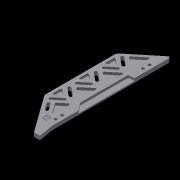
# Autodesk Inventor part: HipShockPlateRight
Saved by Autodesk Inventor 2015 (Build 190159000, 159)
## iProperties
RuleStatus: InUse
Created: 2014-08-28
Part Number: HipShockPlateRight
Material: Generic
Document SubType Name: Modeling
Designer: Inventor
Density: 1 g/cm^3
Appearance: Default
Mass: 78.3969 g
Surface Area: 353.49 cm^2
Volume: 78.3969 cm^3
BeforeDocSave0: UpdateBoundingBox
CX: 66.60 mm
CY: 268.39 mm
CZ: 8.00 mm
Author: Inventor
Autodesk Inventor part; units mm, degrees
ref_plane "YZ Plane" through (0, 0, 0) normal (1, 0, 0) x (0, 1, 0)
ref_plane "XZ Plane" through (0, 0, 0) normal (0, 1, 0) x (-1, 0, 0)
sketch "Base" plane through (0, 0, 0) normal (0, 0, 1) x (1, 0, 0)
  line L0 (6.9563, 266) -> (3.8969, 268.7067)
  line L1 (-54.5437, 220.9056) -> (3.8969, 268.7067)
  line L2 (-54.5437, 220.9056) -> (-54.5437, 75.9056)
  line L3 (0, 0) -> (12.2461, 0)
  line L4 (0, 0) -> (-54.5437, 75.9056)
  line L5 (6.9563, 30) -> (12.2461, 0)
  line L6 (6.9563, 266) -> (6.9563, 30)
  dimension "d1" = 170
  dimension "d3" = 131.5
  dimension "d4" = 99.219
  dimension "d5" = 75.5
  dimension "d6" = 145
  dimension "d7" = 129.281
  dimension "d8" = 144.3
  dimension "d9" = 125.7
  dimension "d10" = 236
  dimension "d11" = 30
  dimension "d15" = 61.5
  constraints: 14 end point, 1 coincident, 1 horizontal, 1 parallel, 1 vertical
  measures "d1" angle of L6 L5
  measures "d3" angle of L0 L6
  measures "d4" angle of L1 L0
  measures "d5" distance of L1.start L0.end
  measures "d6" distance of L1.start L2.end
  measures "d7" angle of L2 L1
  measures "d8" angle of L2 L4
  measures "d9" angle of L4 L3
  measures "d10" distance of L0.start L5.start
  measures "d11" vertical distance of L5.start L3.end
  measures "d15" distance between parallel lines of L6 L2
extrude "BaseFeature" add sketch "Base" along normal blind 8
fillet "BaseFillet1Feature" radius 9 1 edges at (-54.5437, 220.9056, 4)
fillet "BaseFillet2Feature" radius 6 1 edges at (-54.5437, 75.9056, 4)
ref_plane "BaseTopPlane" through (0, 0, 8) normal (0, 0, 1) x (1, 0, 0)
sketch "InsetDetail" plane through (0, 0, 8) normal (0, 0, 1) x (1, 0, 0)
  line L0 (-12.0437, 248.5627) -> (-12.0437, 208.0737)
  line L1 (-12.0437, 208.0737) -> (-36.7942, 228.3182)
  line L2 (-36.7942, 228.3182) -> (-12.0437, 248.5627)
  line L3 (-34.9841, 201.5737) -> (-49.0437, 190.0737)
  line L4 (-49.0437, 213.0737) -> (-34.9841, 201.5737)
  line L5 (-49.0437, 190.0737) -> (-49.0437, 213.0737)
  line L6 (-36.5437, 175.0341) -> (-12.0437, 195.0737)
  line L7 (-12.0437, 195.0737) -> (-12.0437, 154.5847)
  line L8 (-12.0437, 154.5847) -> (-36.5437, 175.0341)
  line L9 (-35.2658, 148.0847) -> (-49.0437, 136.5847)
  line L10 (-49.0437, 159.5847) -> (-35.2658, 148.0847)
  line L11 (-49.0437, 136.5847) -> (-49.0437, 159.5847)
  line L12 (-36.2982, 121.3402) -> (-12.0437, 141.5847)
  line L13 (-12.0437, 141.5847) -> (-12.0437, 101.0957)
  line L14 (-12.0437, 101.0957) -> (-36.2982, 121.3402)
  line L15 (-35.2658, 94.5957) -> (-49.0437, 83.0957)
  line L16 (-49.0437, 106.0957) -> (-35.2658, 94.5957)
  line L17 (-49.0437, 83.0957) -> (-49.0437, 106.0957)
  line L18 (-30.2303, 72.916) -> (-12.0437, 47.6068)
  line L19 (-12.0437, 88.0957) -> (-12.0437, 47.6068)
  line L20 (-30.2303, 72.916) -> (-12.0437, 88.0957)
  line L21 (-5.0437, 98.1402) -> (-5.0437, 194.9501)
  line L22 (6.9563, 196) -> (-5.0437, 194.9501)
  line L23 (6.9563, 83) -> (-5.0437, 98.1402)
  line L24 (6.9563, 30) -> (6.9563, 266) construction
  line L25 (6.9563, 196) -> (6.9563, 83)
  line L26 (-54.5437, 216.6399) -> (-54.5437, 77.8378) construction
  line L27 (3.8969, 268.7067) -> (-51.2419, 223.6064) construction
  line L28 (-53.4162, 74.3365) -> (0, 0) construction
  line L29 (-49.0437, 201.5737) -> (6.9563, 201.5737) construction
  line L30 (-49.0437, 148.0847) -> (6.9563, 148.0847) construction
  line L31 (-49.0437, 94.5957) -> (6.9563, 94.5957) construction
  line L32 (-36.7942, 228.3182) -> (-12.0437, 228.3182) construction
  line L33 (-36.5437, 175.0341) -> (-12.0437, 175.0341) construction
  line L34 (-36.2982, 121.3402) -> (-12.0437, 121.3402) construction
  line L35 (-30.2303, 72.916) -> (-12.0437, 72.916) construction
  dimension "d21" = 95
  dimension "d22" = 141.6
  dimension "d23" = 12
  dimension "d24" = 113
  dimension "d25" = 70
  dimension "d27" = 5.5
  dimension "d29" = 5.5
  dimension "d30" = 5.5
  dimension "d66" = 13
  dimension "d67" = 13
  dimension "d90" = 18
  dimension "d91" = 6.5
  dimension "d93" = 6.5
  dimension "d94" = 6.5
  dimension "d95" = 13
  dimension "d97" = 19
  dimension "d98" = 19
  dimension "d99" = 19
  dimension "d100" = 19
  dimension "d102" = 5.5
  dimension "d105" = 23
  dimension "d106" = 18
  constraints: 64 end point, 16 parallel, 10 point on line, 6 perpendicular, 5 collinear, 5 midpoint, 1 horizontal, 1 vertical
  measures "d21" angle of L22 L21
  measures "d22" angle of L21 L23
  measures "d23" distance between parallel lines of L21 L24
  measures "d24" distance of L23.start L22.start
  measures "d25" distance of L22.start L24.end
  measures "d27" distance between parallel lines of L27 L2
  measures "d29" distance between parallel lines of L26 L11
  measures "d30" distance between parallel lines of L26 L17
  measures "d66" distance of L6.end L0.end
  measures "d67" distance of L12.end L7.end
  measures "d90" distance between parallel lines of L28 L18
  measures "d91" distance from line of L29 L0.end
  measures "d93" distance from line of L30 L7.end
  measures "d94" distance from line of L31 L13.end
  measures "d95" distance of L19.start L13.end
  measures "d97" distance between parallel lines of L24 L0
  measures "d98" distance between parallel lines of L24 L7
  measures "d99" distance between parallel lines of L24 L13
  measures "d100" distance between parallel lines of L24 L19
  measures "d102" distance between parallel lines of L26 L5
  measures "d105" distance of L9.end L10.start
  measures "d106" distance from line of L26 L6.start
extrude "InsetsFeature" cut sketch "InsetDetail" against normal blind 5
fillet "InsetFillet1Feature" radius 3 1 edges at (-5.0437, 194.9501, 5.5)
fillet "InsetFillet2Feature" radius 4 1 edges at (-5.0437, 98.1402, 5.5)
fillet "TriangleInsetFilletsFeature" radius 2 21 edges at (-12.0437, 248.5627, 5.5) (-36.7942, 228.3182, 5.5) (-12.0437, 208.0737, 5.5) (-12.0437, 154.5847, 5.5) (-36.5437, 175.0341, 5.5) (-12.0437, 195.0737, 5.5) (-49.0437, 213.0737, 5.5) (-49.0437, 190.0737, 5.5) (-34.9841, 201.5737, 5.5) (-49.0437, 136.5847, 5.5) (-49.0437, 159.5847, 5.5) (-35.2658, 148.0847, 5.5) (-12.0437, 141.5847, 5.5) (-36.2982, 121.3402, 5.5) (-12.0437, 101.0957, 5.5) (-49.0437, 106.0957, 5.5) (-49.0437, 83.0957, 5.5) (-35.2658, 94.5957, 5.5) (-30.2303, 72.916, 5.5) (-12.0437, 88.0957, 5.5) (-12.0437, 47.6068, 5.5)
sketch "VariableHoles" plane through (0, 0, 8) normal (0, 0, 1) x (1, 0, 0)
  line L0 (-45.7775, 210.4021) -> (-36.8767, 203.1218) construction
  line L1 (-15.31, 210.7453) -> (-34.9015, 226.7701) construction
  line L2 (-36.8767, 200.0256) -> (-45.7775, 192.7453) construction
  line L3 (-34.4587, 122.8757) -> (-15.3253, 138.8457) construction
  line L4 (-45.7621, 103.3567) -> (-37.1054, 96.1312) construction
  line L5 (-15.3253, 103.8348) -> (-34.4587, 119.8048) construction
  line L6 (-37.1054, 93.0603) -> (-45.7621, 85.8348) construction
  line L7 (-28.8022, 74.108) -> (-15.3253, 85.3567) construction
  line L8 (-15.6679, 52.6503) -> (-29.1448, 71.4054) construction
  line L9 (-53.4162, 74.3365) -> (0, 0) construction
  line L10 (-42.1468, 220.0644) -> (-26.6658, 207.4018) construction
  line L11 (6.9563, 30) -> (6.9563, 266) construction
  arc A0 (-28.5652, 205.0797) -> (-24.7665, 209.724) centre (-26.6658, 207.4018) ccw
  arc A1 (-40.2474, 222.3865) -> (-44.0462, 217.7422) centre (-42.1468, 220.0644) ccw
  line L12 (-40.2474, 222.3865) -> (-24.7665, 209.724)
  line L13 (-44.0462, 217.7422) -> (-28.5652, 205.0797)
  line L14 (3.8969, 268.7067) -> (-51.2419, 223.6064) construction
  line L15 (-34.9015, 229.8663) -> (-15.31, 245.8911) construction
  line L16 (-49.0437, 194.2934) -> (-49.0437, 208.854) construction
  line L17 (-49.0437, 201.5737) -> (6.9563, 201.5737) construction
  line L18 (-42.1468, 183.0831) -> (-26.6658, 195.7456) construction
  arc A2 (-24.7665, 193.4235) -> (-28.5652, 198.0677) centre (-26.6658, 195.7456) ccw
  arc A3 (-44.0462, 185.4052) -> (-40.2474, 180.7609) centre (-42.1468, 183.0831) ccw
  line L19 (-40.2474, 180.7609) -> (-24.7665, 193.4235)
  line L20 (-44.0462, 185.4052) -> (-28.5652, 198.0677)
  line L21 (-54.5437, 216.6399) -> (-54.5437, 77.8378) construction
  line L22 (6.9563, 196) -> (6.9563, 83) projected
  line L23 (-54.5437, 148.0847) -> (6.9563, 148.0847) construction
  line L24 (-54.5437, 175.0284) -> (6.9563, 175.0284) construction
  arc A4 (-34.6701, 176.5666) -> (-34.6855, 173.4831) centre (-33.4039, 175.0185) ccw construction
  arc A5 (-40.2474, 169.296) -> (-44.0462, 164.6517) centre (-42.1468, 166.9738) ccw
  line L25 (-44.0462, 164.6517) -> (-28.5652, 151.9891)
  line L26 (-40.2474, 169.296) -> (-24.7665, 156.6334)
  arc A6 (-28.5652, 151.9891) -> (-24.7665, 156.6334) centre (-26.6658, 154.3113) ccw
  line L27 (-42.1468, 166.9738) -> (-26.6658, 154.3113) construction
  arc A7 (-37.1054, 146.5493) -> (-37.1054, 149.6202) centre (-38.387, 148.0847) ccw construction
  line L28 (-44.0462, 131.5178) -> (-28.5652, 144.1803)
  arc A8 (-24.7665, 139.536) -> (-28.5652, 144.1803) centre (-26.6658, 141.8582) ccw
  line L29 (-40.2474, 126.8735) -> (-24.7665, 139.536)
  arc A9 (-44.0462, 131.5178) -> (-40.2474, 126.8735) centre (-42.1468, 129.1956) ccw
  line L30 (-42.1468, 129.1956) -> (-26.6658, 141.8582) construction
  line L31 (-54.5437, 121.3402) -> (6.9563, 121.3402) construction
  arc A10 (-34.4587, 122.8757) -> (-34.4587, 119.8048) centre (-33.1771, 121.3402) ccw construction
  line L32 (-44.0462, 111.1627) -> (-28.5652, 98.5002)
  arc A11 (-40.2474, 115.807) -> (-44.0462, 111.1627) centre (-42.1468, 113.4849) ccw
  line L33 (-40.2474, 115.807) -> (-24.7665, 103.1445)
  arc A12 (-28.5652, 98.5002) -> (-24.7665, 103.1445) centre (-26.6658, 100.8223) ccw
  line L34 (-42.1468, 113.4849) -> (-26.6658, 100.8223) construction
  line L35 (-54.5437, 94.5957) -> (6.9563, 94.5957) construction
  line L36 (6.9563, 30) -> (6.9563, 83) construction
  arc A13 (-37.1054, 93.0603) -> (-37.1054, 96.1312) centre (-38.387, 94.5957) ccw construction
  line L37 (-44.0462, 78.0288) -> (-28.5652, 90.6913)
  arc A14 (-44.0462, 78.0288) -> (-40.2474, 73.3845) centre (-42.1468, 75.7066) ccw
  line L38 (-42.1468, 75.7066) -> (-26.6658, 88.3692) construction
  line L39 (-40.2474, 73.3845) -> (-24.7665, 86.047)
  arc A15 (-24.7665, 86.047) -> (-28.5652, 90.6913) centre (-26.6658, 88.3692) ccw
  line L40 (-37.8435, 62.9469) -> (-29.0904, 50.7656)
  arc A16 (-32.971, 66.4481) -> (-37.8435, 62.9469) centre (-35.4073, 64.6975) ccw
  line L41 (-35.4073, 64.6975) -> (-26.6541, 52.5162) construction
  line L42 (-32.971, 66.4481) -> (-24.2179, 54.2669)
  arc A17 (-29.0904, 50.7656) -> (-24.2179, 54.2669) centre (-26.6541, 52.5162) ccw
  line L43 (-28.8022, 74.108) -> (-44.0855, 61.3515) construction
  point P0 (-35.4039, 175.0284)
  point P1 (-36.387, 148.0847)
  point P2 (-35.1771, 121.3402)
  point P3 (-36.387, 94.5957)
  point P4 (-37.1579, 67.1337)
  dimension "d81" = 19.5555
  dimension "d82" = 9.7777
  dimension "d83" = 20
  dimension "d85" = 6
  dimension "d86" = 6
  dimension "d87" = 5.5
  dimension "d88" = 8.5
  dimension "d112" = 18
  dimension "d113" = 9
  dimension "d114" = 3
  dimension "d115" = 20
  dimension "d116" = 15
  constraints: 54 end point, 40 symmetric about line, 33 point on circle, 15 point on line, 14 centre point, 14 coincident, 7 tangent, 4 parallel, 4 perpendicular, 1 collinear, 1 horizontal, 1 midpoint, 10 other
  measures "d81" distance between parallel lines of L1 L0
  measures "d82" distance between parallel lines of L1 L10
  measures "d83" distance of L10.start L10.end
  measures "d85" diameter of A0
  measures "d86" diameter of A1
  measures "d87" distance between parallel lines of L14 L15
  measures "d88" distance from line of L14 A1.centre
  measures "d112" distance between parallel lines of L9 L8
  measures "d113" distance between parallel lines of L41 L8
  measures "d114" radius of A17
  measures "d115" distance of L38.start L38.end
  measures "d116" distance of L41.start L41.end
extrude "VariableHolesFeature" cut sketch "VariableHoles" against normal through all
sketch "ConnectorHoles" plane through (0, 0, 8) normal (0, 0, 1) x (1, 0, 0)
  line L0 (-1.0437, 234) -> (-1.0437, 45) construction
  line L1 (-5.0437, 99.5332) -> (-5.0437, 192.2011) construction
  line L2 (6.9563, 30) -> (6.9563, 266) construction
  line L3 (0, 0) -> (12.2461, 0) construction
  point P0 (-1.0437, 221)
  point P1 (-1.0437, 58)
  dimension "d118" = 8
  dimension "d119" = 13
  dimension "d120" = 13
  dimension "d131" = 45
  dimension "d134" = 32
  constraints: 2 coincident, 2 end point, 2 point on line, 1 parallel
  measures "d118" distance from line of L2 point (-1.044, 234)
  measures "d119" distance of point (-1.044, 221) L0.start
  measures "d120" distance of L0.end point (-1.044, 58)
  measures "d131" distance from line of L0.end L3
  measures "d134" vertical distance of L0.start L2.end
hole "ConnectorHolesFeature" at (-1.0437, 234, 8) at (-1.0437, 221, 8) at (-1.0437, 58, 8) at (-1.0437, 45, 8) direction (0, 0, -1) diameter 6 end through all
sketch "Logo" plane through (0, 0, 8) normal (0, 0, 1) x (1, 0, 0)
  line L0 (6.9563, 30) -> (6.9563, 83) construction
  line L1 (-10.5437, 35.339) -> (-10.5437, 36.839)
  line L2 (-14.0437, 36.839) -> (-14.0437, 35.339)
  line L3 (-10.5437, 36.839) -> (-14.0437, 36.839)
  line L4 (-16.0437, 42.839) -> (-16.0437, 40.839)
  line L5 (-8.5437, 42.839) -> (-16.0437, 42.839)
  line L6 (-7.5437, 43.839) -> (-17.0437, 43.839)
  line L7 (-16.0437, 32.339) -> (-7.5437, 32.339)
  line L8 (-8.5437, 33.339) -> (-16.0437, 33.339)
  line L9 (-16.0437, 40.839) -> (-8.5437, 40.839)
  line L10 (-16.0437, 38.839) -> (-8.5437, 38.839)
  line L11 (-16.0437, 33.339) -> (-16.0437, 38.839)
  line L12 (-16.0437, 32.339) -> (-16.0437, 33.339)
  line L13 (-16.0437, 33.339) -> (-17.0437, 33.339)
  line L14 (-14.0437, 35.339) -> (-10.5437, 35.339)
  line L15 (-8.5437, 38.839) -> (-8.5437, 33.339)
  line L16 (-8.5437, 40.839) -> (-8.5437, 42.839)
  line L17 (-7.5437, 32.339) -> (-7.5437, 43.839)
  line L18 (-17.0437, 43.839) -> (-17.0437, 33.339)
  dimension "d158" = 2.339
  dimension "d159" = 1
  dimension "d160" = 1
  dimension "d161" = 2
  dimension "d162" = 2
  dimension "d163" = 1
  dimension "d164" = 1
  dimension "d165" = 1
  dimension "d166" = 2
  dimension "d167" = 1
  dimension "d168" = 2
  dimension "d169" = 2
  dimension "d170" = 2
  dimension "d171" = 14.5
  dimension "d172" = 90
  dimension "d174" = 11.5
  dimension "d176" = 3.5
  constraints: 36 end point, 3 parallel, 1 horizontal
  measures "d158" distance from line of L0.start L7
  measures "d159" distance between parallel lines of L7 L8
  measures "d160" distance between parallel lines of L18 L11
  measures "d161" distance between parallel lines of L9 L10
  measures "d162" distance between parallel lines of L5 L9
  measures "d163" distance between parallel lines of L6 L5
  measures "d164" distance between parallel lines of L18 L4
  measures "d165" distance between parallel lines of L17 L16
  measures "d166" distance between parallel lines of L15 L1
  measures "d167" distance between parallel lines of L17 L15
  measures "d168" distance between parallel lines of L8 L14
  measures "d169" distance between parallel lines of L11 L2
  measures "d170" distance between parallel lines of L10 L3
  measures "d171" distance between parallel lines of L0 L17
  measures "d172" angle of L12 L7
  measures "d174" distance between parallel lines of L6 L7
  measures "d176" distance between parallel lines of L1 L2
extrude "LogoFeature" cut sketch "Logo" against normal blind 1
fillet "BaseFillet3Feature" radius 1 4 edges at (12.2461, 0, 4) (0, 0, 4) (6.9563, 266, 4) (3.8969, 268.7067, 4)
equation "\"d29\" = d27"
equation "\"d30\" = d27"
equation "\"d67\" = d66"
body "Solid1"
